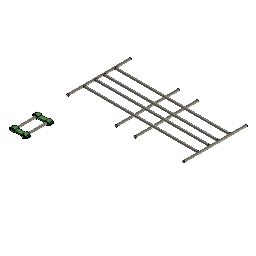
Kerbecs (Autodesk Fusion 360 design; units mm, degrees)
Autodesk Fusion 360 part; units mm, degrees
cylinder "CylinderPrimitive3" add diameter 18 height 736 placed x (0, 0, -1) y (0, 1, 0) z (1, 0, 0) at (0, 0, 0) makes body 1
copy_body "CopyPasteBodies4" bodies 1 makes body 2
move_body "Move2" bodies 2 to x (1, 0, 0) y (0, 1, 0) z (0, 0, 1) at (0, 218, 0)
copy_body "CopyPasteBodies5" bodies 1 2 makes body 3 makes body 4
move_body "Move3" bodies 3 to x (1, 0, 0) y (0, 1, 0) z (0, 0, 1) at (0, 79, 0)
move_body "Move4" bodies 4 to x (1, 0, 0) y (0, 1, 0) z (0, 0, 1) at (0, -79, 0)
cylinder "CylinderPrimitive4" add diameter 18 height 436 placed x (1, 0, 0) y (0, 0, -1) z (0, 1, 0) at (0, 0, 25) separate body makes body 5
move_body "Move5" bodies 5 to x (1, 0, 0) y (0, 1, 0) z (0, 0, 1) at (0, -109, 0)
move_body "Move6" bodies 5 to x (1, 0, 0) y (0, 1, 0) z (0, 0, 1) at (0, 0, -7)
move_body "Move7" bodies 5 to x (1, 0, 0) y (0, 1, 0) z (0, 0, 1) at (9, 0, 0)
copy_body "CopyPasteBodies6" bodies 5 makes body 6
move_body "Move8" bodies 6 to x (1, 0, 0) y (0, 1, 0) z (0, 0, 1) at (318, 0, 0)
copy_body "CopyPasteBodies7" bodies 6 makes body 7
move_body "Move9" bodies 7 to x (1, 0, 0) y (0, 1, 0) z (0, 0, 1) at (132, 0, 0)
copy_body "CopyPasteBodies8" bodies 7 makes body 8
move_body "Move10" bodies 8 to x (1, 0, 0) y (0, 1, 0) z (0, 0, 1) at (318, 0, 0)
move_face "OffsetFaces1" offset 50 1 faces at (736, 0.3267, 5.1676) on bodies 1
move_face "OffsetFaces2" offset 50 1 faces at (736, 79.3267, 5.1676) on bodies 3
move_face "OffsetFaces3" offset 50 1 faces at (736, 141.3455, -1.8705) on bodies 4
move_face "OffsetFaces4" offset 50 1 faces at (736, 220.3455, -1.8705) on bodies 2
move_body "Move11" bodies 5 to x (1, 0, 0) y (0, 1, 0) z (0, 0, 1) at (-18, 0, 0)
move_body "Move12" bodies 5 to x (1, 0, 0) y (0, 1, 0) z (0, 0, 1) at (0, 0, -18)
move_body "Move13" bodies 8 to x (1, 0, 0) y (0, 1, 0) z (0, 0, 1) at (18, 0, -18)
move_body "Move14" bodies 6 7 to x (1, 0, 0) y (0, 1, 0) z (0, 0, 1) at (0, 0, -36)
cylinder "CylinderPrimitive5" add diameter 18 height 200 placed x (1, 0, 0) y (0, 0, -1) z (0, 1, 0) at (0, 0, -75) separate body makes body 9
move_body "Move16" bodies 9 to x (1, 0, 0) y (0, 1, 0) z (0, 0, 1) at (0, -500, 0)
move_body "Move17" bodies 9 to x (1, 0, 0) y (0, 1, 0) z (0, 0, 1) at (0, 0, 75)
move_body "Move18" bodies 9 to x (1, 0, 0) y (0, 0.573576, 0.819152) z (0, -0.819152, 0.573576) at (0, -220.5842, 405.7382)
copy_body "CopyPasteBodies10" bodies 9 makes body 10
move_body "Move19" bodies 10 to x (1, 0, 0) y (0, 1, 0) z (0, 0, 1) at (75, 0, 0)
move_body "Move20" bodies 9 to x (1, 0, 0) y (0, 0.573576, -0.819152) z (0, 0.819152, 0.573576) at (0, -212.1269, -425.492)
move_body "Move21" bodies 10 to x (1, 0, 0) y (0, 0.573576, -0.819152) z (0, 0.819152, 0.573576) at (0, -212.1269, -425.492)
sketch "Sketch8" plane through (0, -506.2875, 0) normal (0, -1, 0) x (1, 0, 0)
  circle A0 centre (0, -12.0782) radius 9
  circle A1 centre (0, -12.0782) radius 9
  line L0 (-13.0767, -7.0782) -> (-23.0767, -7.0782)
  line L1 (-23.0767, -7.0782) -> (-23.0767, -11.0782)
  line L2 (-23.0767, -11.0782) -> (-13.9642, -11.0782)
  line L3 (-13.0767, -17.0782) -> (-23.0767, -17.0782)
  line L4 (-23.0767, -17.0782) -> (-23.0767, -13.0782)
  line L5 (-23.0767, -13.0782) -> (-13.9642, -13.0782)
  arc A2 (-13.0767, -17.0782) -> (13.0767, -17.0782) centre (0, -12.0782) ccw
  arc A3 (13.0767, -7.0782) -> (-13.0767, -7.0782) centre (0, -12.0782) ccw
  line L6 (13.0767, -7.0782) -> (37.5, -7.0782)
  line L7 (13.0767, -17.0782) -> (37.5, -17.0782)
  line L8 (-13.9642, -11.0782) -> (-8.9443, -11.0782)
  line L9 (-13.9642, -13.0782) -> (-8.9443, -13.0782)
  line L10 (98.0767, -11.0782) -> (88.9642, -11.0782)
  line L11 (98.0767, -17.0782) -> (98.0767, -13.0782)
  line L12 (88.0767, -17.0782) -> (98.0767, -17.0782)
  circle A4 centre (75, -12.0782) radius 9
  line L13 (98.0767, -13.0782) -> (88.9642, -13.0782)
  line L14 (61.9233, -17.0782) -> (37.5, -17.0782)
  line L15 (61.9233, -7.0782) -> (37.5, -7.0782)
  arc A5 (88.0767, -7.0782) -> (61.9233, -7.0782) centre (75, -12.0782) ccw
  line L16 (88.0767, -7.0782) -> (98.0767, -7.0782)
  line L17 (88.9642, -13.0782) -> (83.9443, -13.0782)
  arc A6 (61.9233, -17.0782) -> (88.0767, -17.0782) centre (75, -12.0782) ccw
  line L18 (88.9642, -11.0782) -> (83.9443, -11.0782)
  circle A7 centre (75, -12.0782) radius 9
  line L19 (98.0767, -7.0782) -> (98.0767, -11.0782)
  point P0 (75, 0)
  dimension "d85" = 18
  dimension "d86" = 28
  dimension "d90" = 10
  dimension "d91" = 4
  dimension "d92" = 4
  constraint concentric A0 A1
  constraint concentric A1 A2
  constraint coincident A3.start A2
  constraint horizontal L0
  constraint perpendicular L0 L1
  constraint perpendicular L1 L2
  constraint perpendicular L1 L3
  constraint perpendicular L3 L4
  constraint perpendicular L4 L5
  constraint concentric A2 A3
  constraint coincident A1 L8.end
  constraint parallel L2 L8
  constraint coincident A1 L9.end
  constraint parallel L5 L9
  measures "d85" diameter of A1
  measures "d86" diameter of A2
  measures "d90" distance of L0.start L0.end
  measures "d91" distance of L0.end L1.end
  measures "d92" distance of L3.end L4.end
extrude "Extrude4" add sketch "Sketch8" along normal blind 30 separate body contours A0 A1 L0 L1 L2 L3 L4 L5 A2 A3 L6 L7 L8 L9 L10 L11 L12 A4 L13 L14 L15 A5 L16 L17 A6 L18 A7 L19 makes body 11
move_body "Move23" bodies 11 to x (1, 0, 0) y (0, 1, 0) z (0, 0, 1) at (0, -35, 0)
copy_body "CopyPasteBodies11" bodies 11 makes body 12
move_body "Move24" bodies 12 to x (1, 0, 0) y (0, 1, 0) z (0, 0, 1) at (0, -60, 0)
move_body "Move25" bodies 11 to x (1, 0, 0) y (0, 1, 0) z (0, 0, 1) at (0, 230, 0)
move_body "Move26" bodies 12 to x (1, 0, 0) y (0, 1, 0) z (0, 0, 1) at (0, 130, 0)
cylinderprimitive "CylinderPrimitive2" [suppressed]
equation "d11 = 18.00 mm + 200 mm"
equation "d14 = ( ( 18 + 200 ) / 2 ) * 1 mm - 30 mm"
equation "d17 = -( ( ( 18 + 200 ) / 2 ) * 1 mm - 30 mm )"
equation "d33 = 114 mm + 18 mm"
named bodies: "Pipe 1", "Pipe 4", "Pipe 1 (1)", "Pipe 1 (1) (1)", "Pipe 2", "Pipe 3", "Pipe 5", "Pipe 6", "Pipe 5 (1)", "Pipe 7", "Pipe 5 (1) (1)", "Pipe8", "Thigh 1", "Thigh 2", "Thigh Clamp 1", "Thigh Clamp 2"
